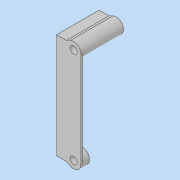
# Autodesk Inventor part: ArduinoNanoHolder
Saved by Autodesk Inventor 2017 (Build 210142000, 142)
## iProperties
Created: 2017-04-15
Part Number: ArduinoNanoHolder
Material: Generic
Document SubType Name: Modeling
Designer: Derek Wider
Mass: 1.02199 g
Surface Area: 19.3795 cm^2
Volume: 1.02199 cm^3
Density: 1 g/cm^3
Appearance: Default
Author: Derek Wider
Autodesk Inventor part; units mm, degrees
ref_plane "YZ Plane" through (0, 0, 0) normal (1, 0, 0) x (0, 1, 0)
ref_plane "XZ Plane" through (0, 0, 0) normal (0, 1, 0) x (-1, 0, 0)
ref_plane "XY Plane" through (0, 0, 0) normal (0, 0, 1) x (1, 0, 0)
sketch "Sketch1" plane through (0, 0, 0) normal (0, 0, 1) x (1, 0, 0)
  circle A0 centre (36.2951, 20.955) radius 1.5875
  circle A1 centre (36.2951, 20.955) radius 3.175
  line L0 (0, 0) -> (36.2951, 20.955)
  line L1 (0, 0) -> (38.1631, 0)
  circle A2 centre (36.2951, -20.955) radius 1.5875
  circle A3 centre (36.2951, -20.955) radius 3.175
  line L2 (28.8021, 22.9235) -> (30.0721, 22.9235)
  line L3 (30.0721, 22.9235) -> (30.0721, 20.1295)
  line L4 (30.0721, 20.1295) -> (28.8021, 20.1295)
  line L5 (28.8021, 20.1295) -> (28.8021, 22.9235)
  line L6 (30.0721, 22.9235) -> (31.8501, 22.9235)
  line L7 (31.8501, 22.9235) -> (31.8501, 21.6535)
  line L8 (31.8501, 21.6535) -> (30.0721, 21.6535)
  line L9 (30.0721, 21.6535) -> (30.0721, 22.9235)
  line L10 (31.8501, 22.9235) -> (33.1201, 22.9235)
  line L11 (33.1201, 22.9235) -> (33.1201, 20.1295)
  line L12 (33.1201, 20.1295) -> (31.8501, 20.1295)
  line L13 (31.8501, 20.1295) -> (31.8501, 22.9235)
  line L14 (33.1201, 22.9235) -> (34.8833, 23.7988)
  line L15 (30.0721, -21.6535) -> (31.8501, -21.6535)
  line L16 (31.8501, -21.6535) -> (31.8501, -22.9235)
  line L17 (31.8501, -22.9235) -> (30.0721, -22.9235)
  line L18 (30.0721, -22.9235) -> (30.0721, -21.6535)
  line L19 (28.8021, -20.1295) -> (30.0721, -20.1295)
  line L20 (30.0721, -20.1295) -> (30.0721, -22.9235)
  line L21 (30.0721, -22.9235) -> (28.8021, -22.9235)
  line L22 (28.8021, -22.9235) -> (28.8021, -20.1295)
  line L23 (31.8501, -22.9235) -> (33.1201, -22.9235)
  line L24 (33.1201, -22.9235) -> (33.1201, -20.1295)
  line L25 (33.1201, -20.1295) -> (31.8501, -20.1295)
  line L26 (31.8501, -20.1295) -> (31.8501, -22.9235)
  line L27 (33.1201, 20.1295) -> (33.5222, 19.4085)
  line L28 (33.1201, -20.1295) -> (33.5222, -19.4085)
  line L29 (33.1201, -22.9235) -> (34.8833, -23.7988)
  dimension "d0" = 3.175
  dimension "d1" = 6.35
  dimension "d2" = 41.91
  dimension "d3" = 30
  dimension "d4" = 1.27
  dimension "d5" = 1.27
  dimension "d6" = 1.778
  dimension "d7" = 1.27
  dimension "d8" = 2.794
  dimension "d9" = 1.27
  dimension "d10" = 1.27
  dimension "d11" = 1.778
  dimension "d12" = 2.794
  dimension "d13" = 1.27
  dimension "d14" = 43.307
  dimension "d15" = 0.6985
  constraints: 60 end point, 12 parallel, 7 horizontal, 6 perpendicular, 6 tangent, 4 centre point, 4 point on circle, 2 coincident, 2 point on line, 2 symmetric about line, 2 other
  measures "d0" diameter of A0
  measures "d1" diameter of A1
  measures "d2" distance of L0.start L0.end
  measures "d3" angle of L0 L1
  measures "d4" distance of L2.start L2.end
  measures "d5" distance of L6.end L10.end
  measures "d6" distance of L2.end L6.end
  measures "d7" distance between parallel lines of L6 L8
  measures "d8" distance between parallel lines of L2 L4
  measures "d9" distance between parallel lines of L20 L22
  measures "d10" distance between parallel lines of L26 L24
  measures "d11" distance of L16.end L17.end
  measures "d12" distance between parallel lines of L21 L19
  measures "d13" distance between parallel lines of L17 L15
  measures "d14" distance between parallel lines of L15 L8
  measures "d15" distance from line of A3.centre L15
extrude "Extrusion1" add sketch "Sketch1" against normal blind 18.0086 contours A1 | A1 L11 L14 | L11 L12 L13 L7 L10 | A1 L27 L11 | L7 L8 L3 L6 | L3 L4 L5 L2
extrude "Extrusion2" add sketch "Sketch1" against normal blind 3.175 contours A3 | A3 L24 L28 | L29 L24 A3 | L24 L23 L16 L26 L25 | L17 L18 L15 L16 | L21 L22 L19 L20 L18
sketch "Sketch2" plane through (0, 0, 0) normal (0, 0, 1) x (1, 0, 0)
  circle A0 centre (36.2951, 20.955) radius 1.5875 projected
  line L0 (30.0721, 21.6535) -> (31.8501, 21.6535) projected
  line L1 (31.8501, 21.6535) -> (31.8501, 20.1295) projected
  line L2 (31.8501, 20.1295) -> (33.1201, 20.1295) projected
  line L3 (33.1201, 20.1295) -> (33.5222, 19.4085) projected
  arc A1 (33.5222, 19.4085) -> (34.8833, 23.7988) centre (36.2951, 20.955) ccw projected
  line L4 (34.8833, 23.7988) -> (33.1201, 22.9235) projected
  line L5 (33.1201, 22.9235) -> (28.8021, 22.9235) projected
  line L6 (28.8021, 22.9235) -> (28.8021, 20.1295) projected
  line L7 (28.8021, 20.1295) -> (30.0721, 20.1295) projected
  line L8 (30.0721, 20.1295) -> (30.0721, 21.6535) projected
  circle A2 centre (36.2951, -20.955) radius 1.5875 projected
  line L9 (28.8021, -22.9235) -> (33.1201, -22.9235) projected
  line L10 (33.1201, -22.9235) -> (34.8833, -23.7988) projected
  arc A3 (34.8833, -23.7988) -> (33.5222, -19.4085) centre (36.2951, -20.955) ccw projected
  line L11 (33.5222, -19.4085) -> (33.1201, -20.1295) projected
  line L12 (33.1201, -20.1295) -> (31.8501, -20.1295) projected
  line L13 (31.8501, -20.1295) -> (31.8501, -21.6535) projected
  line L14 (31.8501, -21.6535) -> (30.0721, -21.6535) projected
  line L15 (30.0721, -21.6535) -> (30.0721, -20.1295) projected
  line L16 (30.0721, -20.1295) -> (28.8021, -20.1295) projected
  line L17 (28.8021, -20.1295) -> (28.8021, -22.9235) projected
  line L18 (28.8021, 20.1295) -> (28.8021, -20.1295)
  line L19 (39.4701, 20.955) -> (39.4701, -20.955)
  point P0 (0, 0)
  constraints: 4 end point, 2 point on circle, 1 tangent, 1 vertical
extrude "Extrusion3" add sketch "Sketch2" along normal blind 0.635
equation "\"d15\" = -0.5 * d2 + 0.5 * d14"
body "Solid1"
